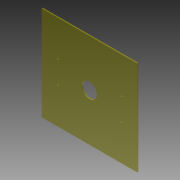
# Autodesk Inventor part: visor
Saved by Autodesk Inventor 2014 SP2 (Build 180246200, 246)
## iProperties
Created: 2016-05-05
Part Number: visor
Material: Generic
Document SubType Name: Modeling
Designer: cruiser
Density: 1 g/cm^3
Appearance: Clear - Yellow
Author: cruiser
Autodesk Inventor part; units mm, degrees
ref_plane "YZ Plane" through (0, 0, 0) normal (1, 0, 0) x (0, 1, 0)
ref_plane "XZ Plane" through (0, 0, 0) normal (0, 1, 0) x (-1, 0, 0)
ref_plane "XY Plane" through (0, 0, 0) normal (0, 0, 1) x (1, 0, 0)
sketch "Sketch1" plane through (0, 0, 0) normal (0, 1, 0) x (-1, 0, 0)
  line L0 (126.9625, -125.6) -> (-126.9625, -125.6)
  line L1 (-126.9625, -125.6) -> (-126.9625, 125.6)
  line L2 (-126.9625, 125.6) -> (126.9625, 125.6)
  line L3 (126.9625, 125.6) -> (126.9625, -125.6)
  line L4 (126.9625, -125.6) -> (-126.9625, 125.6) construction
  line L5 (-126.9625, -125.6) -> (126.9625, 125.6) construction
  point P0 (0, 0)
  dimension "d0" = 253.925
  dimension "d1" = 251.2
  constraints: 12 end point, 2 midpoint, 2 parallel, 1 horizontal, 1 perpendicular
  measures "d0" distance of L1.end L2.end
  measures "d1" distance of L0.end L1.end
extrude "Extrusion1" add sketch "Sketch1" along normal blind 3.15
sketch "Sketch4" plane through (0, 0, 0) normal (0, -1, 0) x (1, 0, 0)
  line L0 (-126.9625, 125.6) -> (-126.9625, -125.6) projected
  line L1 (126.9625, -40) -> (-126.9625, -40)
  line L2 (-126.9625, -40) -> (-126.9625, 40)
  line L3 (-126.9625, 40) -> (126.9625, 40)
  line L4 (126.9625, 40) -> (126.9625, -40)
  line L5 (126.9625, -40) -> (-126.9625, 40) construction
  line L6 (-126.9625, -40) -> (126.9625, 40) construction
  circle A0 centre (-84.6417, 30) radius 2.5
  line L7 (0, 0) -> (-126.9625, 0)
  line L8 (-126.9625, 0) -> (-126.9625, 40)
  line L9 (-126.9625, 40) -> (0, 40)
  line L10 (0, 40) -> (0, 0)
  circle A1 centre (-84.6417, -30) radius 2.5
  circle A2 centre (84.6417, 30) radius 2.5
  circle A3 centre (84.6417, -30) radius 2.5
  circle A4 centre (0, 0) radius 20
  dimension "d20" = 80
  dimension "d21" = 5
  dimension "d22" = 10
  dimension "d23" = 84.6417
  dimension "d24" = 40
  constraints: 20 end point, 5 centre point, 4 parallel, 3 symmetric about line, 2 horizontal, 2 midpoint, 2 perpendicular, 1 coincident, 1 point on line, 3 other
  measures "d20" distance of L1.end L2.end
  measures "d21" diameter of A0
  measures "d22" distance from line of L3 A0.centre
  measures "d23" distance from line of L10 A0.centre
  measures "d24" diameter of A4
extrude "Extrusion4" cut sketch "Sketch4" against normal up to next contours A4 L10 L7 | L7 L10 A4 | A0 | A1 | A2 | A3
equation "\"d0\" = visor_x"
equation "\"d1\" = 2 * visor_y + frame_y"
equation "\"d2\" = clear_acrylic"
equation "\"d20\" = frame_y"
equation "\"d21\" = m5_diameter"
equation "\"d22\" = 0.5 * visor_overlap"
equation "\"d23\" = 0.333333 * visor_x"
equation "\"d24\" = 0.5 * frame_y"
equation "\"sm_thickness\" = 1.5875"
equation "\"very_thick_acrylic\" = 9.45"
equation "\"thick_acrylic\" = 5.88"
equation "\"thin_acrylic\" = 3.15"
equation "\"clear_acrylic\" = 3.15"
equation "\"wood_thickness\" = 6.72"
equation "\"m3_diameter\" = 3"
equation "\"m4_diameter\" = 4"
equation "\"m5_diameter\" = 5"
equation "\"brass_insert_drill\" = 4"
equation "\"m5_brass_insert_drill\" = 6.7"
equation "\"m3_main_length\" = 14"
equation "\"m3_main_nut_width\" = 5.7"
equation "\"m3_main_nut_thickness\" = 2.5"
equation "\"m3_main_extra\" = 1"
equation "\"stepper_screw_space\" = 35"
equation "\"stepper_shaft_diameter\" = 5"
equation "\"stepper_body_diameter\" = 28"
equation "\"laser_body_diameter\" = 12"
equation "\"t_carrier\" = 5.88"
equation "\"t_wall\" = 5.88"
equation "\"t_window\" = 3.15"
equation "\"carrier_y\" = 251"
equation "\"carrier_z\" = 12"
equation "\"carrier_z2\" = 25"
equation "\"protection_slot\" = 44.2"
equation "\"protection_slot_offset\" = 55.25"
equation "\"window_z\" = 332.225"
equation "\"window_y\" = 93.75"
equation "\"door_sensor\" = 35"
equation "\"reservoir_x\" = 201"
equation "\"reservoir_y\" = 201"
equation "\"linear_bearing_spacing\" = 271"
equation "\"motor_spacing\" = 337"
equation "\"t_tray\" = 3.15"
equation "\"tray_border\" = 25"
equation "\"tray_x\" = 251"
equation "\"tray_y\" = 251"
equation "\"bed_z\" = 25"
equation "\"brass_keep_out\" = 8"
equation "\"tape_keep_out\" = 2"
equation "\"tape_thickness\" = 2"
equation "\"t_crane\" = 6.72"
equation "\"crane_z2\" = 12"
equation "\"end_stop_spacing\" = 19"
equation "\"thumb_nut_offset_y\" = 0"
equation "\"thumb_nut_diameter\" = 7"
equation "\"z_min_from_center\" = 115"
equation "\"t_frame\" = 6.72"
equation "\"frame_top_z\" = 385"
equation "\"frame_bottom_z\" = 275"
equation "\"frame_total_z\" = 661.5875"
equation "\"frame_y\" = 80"
equation "\"frame_border\" = 48.0375"
equation "\"frame_foot_z\" = 12"
equation "\"frame_tilt\" = 1deg"
equation "\"printer_z\" = 289"
equation "\"lcd_x\" = 72"
equation "\"lcd_y\" = 25"
equation "\"subframe_x\" = 66"
equation "\"subframe_y_offset\" = 27.5"
equation "\"laser_y_offset\" = 19.4"
equation "\"laser_diameter\" = 12"
equation "\"laser_z_offset\" = 55"
equation "\"laser_y\" = 15"
equation "\"laser_z\" = 75"
equation "\"t_galvo_frame\" = 6.72"
equation "\"galvo_frame_x\" = 66"
equation "\"galvo_frame_z\" = 65"
equation "\"galvo_frame_y_offset\" = 27.5"
equation "\"drawer_x\" = 257.3"
equation "\"drawer_y\" = 90.3375"
equation "\"drawer_z\" = 278.175"
equation "\"drawer_z_from_bottom\" = 25"
equation "\"nema17_x\" = 43"
equation "\"visor_y\" = 85.6"
equation "\"visor_x\" = 253.925"
equation "\"door_z\" = 332.225"
equation "\"door_x\" = 251"
equation "\"window_overlap\" = 48"
equation "\"door_overlap\" = 48"
equation "\"acrylic_into_frame\" = 5"
equation "\"m3_press_nut_drill\" = 4.5"
equation "\"m3_head\" = 6"
equation "\"m5_head\" = 10.3"
equation "\"m5_press_nut_drill\" = 6.5"
equation "\"drawer_support_from_top\" = 48"
equation "\"laser_gap\" = 1"
equation "\"frame_screw_from_center\" = 25"
equation "\"drawer_screw_from_center\" = 55"
equation "\"frame_face_y\" = 45"
equation "\"switch_spacing\" = 19"
equation "\"subframe_y\" = 55"
equation "\"al_thickness\" = 1.5875"
equation "\"rivet_diameter\" = 3.3"
equation "\"bend_factor\" = 2.26205"
equation "\"al_bend\" = 3.591"
equation "\"sm_bend\" = 3.591"
equation "\"frame_x\" = 353.375"
equation "\"carrier_y2\" = 76.825"
equation "\"visor_overlap\" = 20"
body "Solid1"
